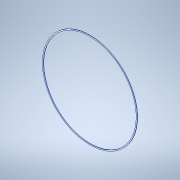
# Autodesk Inventor part: Уплотнение фонарь
Saved by Autodesk Inventor 2021 (Build 250183000, 183)
## iProperties
Created: 2020-12-08
Part Number: Уплотнение фонарь
Material: Алюминий 6061
Document SubType Name: Modeling
Designer: Тимоха
Mass: 38.5945 g
Surface Area: 200.119 cm^2
Volume: 14.2942 cm^3
Density: 2.7 g/cm^3
Appearance: Алюминий — плоский
Author: Тимоха
Autodesk Inventor part; units mm, degrees
ref_plane "YZ Plane" through (0, 0, 0) normal (1, 0, 0) x (0, 1, 0)
ref_plane "XZ Plane" through (0, 0, 0) normal (0, 1, 0) x (-1, 0, 0)
ref_plane "XY Plane" through (0, 0, 0) normal (0, 0, 1) x (1, 0, 0)
sketch "Эскиз1" plane through (0, 0, 0) normal (0, 0, 1) x (1, 0, 0)
  circle A0 centre (0, 0) radius 230
  circle A1 centre (0, 0) radius 225
  dimension "d0" = 460
  dimension "d1" = 450
  constraints: 2 centre point, 2 coincident
  measures "d0" diameter of A0
  measures "d1" diameter of A1
extrude "Выдавливание1" add sketch "Эскиз1" along normal blind 2
